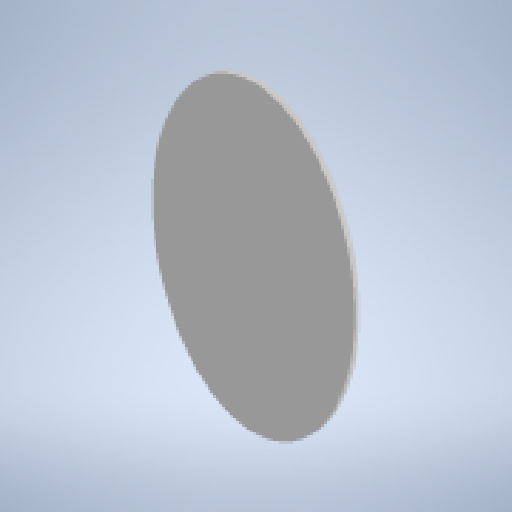
# Autodesk Inventor part: нижний эллипс тела
Saved by Autodesk Inventor 2023.1 (Build 271208000, 208)
## iProperties
Created: 2024-11-21
Part Number: нижний эллипс тела
Material: Типовые
Document SubType Name: Modeling
Designer: DELL
Density: 1 g/cm^3
Appearance: По умолчанию
Author: DELL
Autodesk Inventor part; units mm, degrees
ref_plane "YZ Plane" through (0, 0, 0) normal (1, 0, 0) x (0, 1, 0)
ref_plane "XZ Plane" through (0, 0, 0) normal (0, 1, 0) x (-1, 0, 0)
ref_plane "XY Plane" through (0, 0, 0) normal (0, 0, 1) x (1, 0, 0)
sketch "Эскиз1" plane through (0, 0, 0) normal (0, 0, 1) x (1, 0, 0)
  line L0 (2.6725, 99.2298) -> (22.6725, -99.2298) construction
  ellipse E0 centre (12.6725, 0) end of major axis (12.6725, -120) minor radius 80
  dimension "d2" = 120
  dimension "d3" = 80
  constraints: 2 end point, 1 midpoint, 4 other
extrude "Выдавливание1" add sketch "Эскиз1" against normal blind 4
